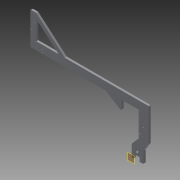
# Autodesk Inventor part: Left Climber Hook_v2
Saved by Autodesk Inventor 2013 (Build 170138000, 138)
## iProperties
Created: 2013-03-16
Part Number: Left Climber Hook_v2
Material: Generic
Document SubType Name: Modeling
Designer: Arpan
Density: 1 g/cm^3
Author: Arpan
Autodesk Inventor part; units mm, degrees
ref_plane "YZ Plane" through (0, 0, 0) normal (1, 0, 0) x (0, 1, 0)
ref_plane "XZ Plane" through (0, 0, 0) normal (0, 1, 0) x (-1, 0, 0)
ref_plane "XY Plane" through (0, 0, 0) normal (0, 0, 1) x (1, 0, 0)
sketch "Sketch1" plane through (0, 0, 0) normal (0, 0, 1) x (1, 0, 0)
  line L0 (0, 0) -> (6.35, 0)
  line L1 (6.35, 0) -> (6.35, 12.7)
  line L2 (6.35, 12.7) -> (25.4, 12.7)
  line L3 (25.4, 12.7) -> (25.4, 0)
  line L4 (25.4, 0) -> (31.75, 0)
  circle A0 centre (15.875, 25.4) radius 4.7815
  line L5 (-323.85, 246.5917) -> (-305.435, 246.5917)
  line L6 (-323.85, 142.875) -> (-83.185, 142.875)
  line L7 (-83.185, 142.875) -> (-37.2427, 114.1611)
  line L8 (-32.385, 142.875) -> (22.225, 142.875)
  line L9 (-32.385, 116.8535) -> (-32.385, 142.875)
  arc A1 (-37.2427, 114.1611) -> (-32.385, 116.8535) centre (-35.56, 116.8535) ccw
  line L10 (-323.85, 168.275) -> (-323.85, 246.5917)
  line L11 (-323.85, 246.5917) -> (-304.8, 246.5917)
  line L12 (-304.8, 229.8394) -> (-304.8, 168.275)
  line L13 (-323.85, 168.275) -> (-323.85, 142.875)
  line L14 (0, 0) -> (0, 38.1)
  line L15 (53.975, -21.4734) -> (53.975, 330.2514) construction
  line L16 (0, 38.1) -> (22.225, 63.5)
  line L17 (22.225, 63.5) -> (22.225, 142.875)
  line L18 (53.975, 63.5) -> (53.975, 168.275)
  line L19 (53.975, 63.5) -> (53.975, 168.275)
  line L20 (22.225, 63.5) -> (22.225, 142.875)
  line L21 (-32.385, 142.875) -> (22.225, 142.875)
  line L22 (-83.185, 142.875) -> (-323.85, 142.875)
  line L23 (31.75, 0) -> (38.1, 0)
  line L24 (38.1, 0) -> (38.1, 38.1)
  line L25 (38.1, 38.1) -> (53.975, 63.5)
  line L26 (38.1, 0) -> (31.75, 0)
  line L27 (-304.8, 246.5917) -> (-213.7569, 168.275)
  line L28 (-233.2314, 168.275) -> (-304.8, 229.8394)
  line L29 (53.975, 168.275) -> (-213.7569, 168.275)
  line L30 (-233.2314, 168.275) -> (-304.8, 168.275)
  line L31 (-304.8, 168.275) -> (-233.2314, 168.275)
  line L32 (-213.7569, 168.275) -> (53.975, 168.275)
  circle A2 centre (-285.75, 149.225) radius 1.5875
  circle A3 centre (-285.75, 161.925) radius 1.5875
  point P0 (-32.385, 111.125)
  point P1 (-359.41, 168.275)
  dimension "d0" = 6.35
  dimension "d1" = 12.7
  dimension "d2" = 19.05
  dimension "d3" = 6.35
  dimension "d4" = 12.7
  dimension "d5" = 9.5631
  dimension "d6" = 12.7
  dimension "d8" = 377.825
  dimension "d17" = 103.7167
  dimension "d19" = 9.525
  dimension "d25" = 31.75
  dimension "d26" = 3.175
  dimension "d27" = 50.8
  dimension "d30" = 19.05
  dimension "d63" = 38.1
  dimension "d68" = 0
  dimension "d69" = 54.61
  dimension "d71" = 22.225
  dimension "d72" = 0
  dimension "d74" = 79.375
  dimension "d75" = 78.3167
  dimension "d76" = 240.665
  dimension "d87" = 6.35
  dimension "d88" = 38.1
  dimension "d89" = 25.4
  dimension "d91" = 25.4
  dimension "d94" = 12.7
  dimension "d95" = 19.05
  dimension "d96" = 25.4
  dimension "d97" = 40.703
  dimension "d98" = 267.7319
  dimension "d109" = 3.175
  dimension "d110" = 3.175
  dimension "d111" = 38.1
  dimension "d112" = 38.1
  dimension "d113" = 6.35
  dimension "d114" = 6.35
  constraints: 66 end point, 10 perpendicular, 9 parallel, 4 centre point, 4 collinear, 4 point on line, 3 horizontal, 2 point on circle, 2 tangent, 2 vertical
  measures "d0" distance of L0.start L0.end
  measures "d1" distance of L0.end L1.end
  measures "d2" distance of L1.end L2.end
  measures "d3" distance of L3.end L4.end
  measures "d4" distance of L2.end L3.end
  measures "d5" diameter of A0
  measures "d6" distance from line of L2 A0.centre
  measures "d8" distance of L29.start L10.start
  measures "d17" distance of L6.start L5.start
  measures "d19" distance from line of L3 A0.centre
  measures "d25" distance of L8.start point (-32.385, 111.125)
  measures "d26" radius of A1
  measures "d27" distance from line of L9 L6.end
  measures "d30" distance of L5.start L11.end
  measures "d63" distance of L0.start L14.end
  measures "d68" distance of L17.end L8.end
  measures "d69" distance of L8.start L8.end
  measures "d71" distance from line of L14 L16.end
  measures "d72" distance of L29.start L18.end
  measures "d74" distance of L16.end L17.end
  measures "d75" distance of L12.end L11.end
  measures "d76" distance of L6.start L6.end
  measures "d87" distance of L4.end L23.end
  measures "d88" distance of L23.end L24.end
  measures "d89" vertical distance of L14.end L16.end
  measures "d91" vertical distance of L18.start L24.end
  measures "d94" distance between parallel lines of L28 L27
  measures "d95" distance between parallel lines of L10 L12
  measures "d96" distance between parallel lines of L6 L30
  measures "d97" angle of L30 L28
  measures "d98" distance of L29.start L27.end
  measures "d109" diameter of A2
  measures "d110" diameter of A3
  measures "d111" distance from line of L13 A3.centre
  measures "d112" distance from line of L13 A2.centre
  measures "d113" distance from line of L6 A2.centre
  measures "d114" distance from line of L30 A3.centre
ref_plane "Work Plane4" through (0, 0, 9.525) normal (0, 0, 1) x (1, 0, 0)
ref_plane "Work Plane3" through (0, 0, 9.525) normal (0, 0, 1) x (1, 0, 0)
extrude "Extrusion9" add sketch "Sketch1" along normal blind 6.35 contours L14 L16 L17 L8 L9 A1 L7 L6 L13 L10 L5 L11 L27 L29 L18 L25 L24 L23 L4 L3 L2 L1 L0 | A2 | A3
sketch "Sketch8" plane through (0, 0, 6.35) normal (0, 0, 1) x (1, 0, 0)
  line L0 (-304.8, 246.5917) -> (-323.85, 246.5917) projected
  line L1 (-323.85, 246.5917) -> (-323.85, 142.875) projected
  circle A0 centre (-309.2958, 218.3215) radius 1.905
  circle A1 centre (-319.405, 195.3091) radius 1.905
  dimension "d101" = 3.81
  dimension "d102" = 3.81
  dimension "d103" = 14.5542
  dimension "d104" = 28.2702
  dimension "d105" = 4.445
  dimension "d106" = 51.2826
  constraints: 2 centre point
  measures "d101" diameter of A0
  measures "d102" diameter of A1
  measures "d103" distance from line of L1 A0.centre
  measures "d104" distance from line of L0 A0.centre
  measures "d105" distance from line of L1 A1.centre
  measures "d106" distance from line of A1.centre L0
extrude "Extrusion10" cut sketch "Sketch8" against normal blind 6.35
sketch "Sketch9" plane through (0, 0, 6.35) normal (0, 0, 1) x (1, 0, 0)
  line L0 (-323.85, 246.5917) -> (-323.85, 142.875) projected
  line L1 (-323.85, 142.875) -> (-83.185, 142.875) projected
  circle A0 centre (-285.75, 155.575) radius 1.5875
  circle A1 centre (-285.75, 147.6375) radius 1.5875
  dimension "d115" = 3.175
  dimension "d116" = 3.175
  dimension "d117" = 38.1
  dimension "d118" = 38.1
  dimension "d119" = 4.7625
  dimension "d124" = 7.9375
  constraints: 2 centre point
  measures "d115" diameter of A0
  measures "d116" diameter of A1
  measures "d117" distance from line of L0 A0.centre
  measures "d118" distance from line of L0 A1.centre
  measures "d119" distance from line of L1 A1.centre
  measures "d124" distance of A1.centre A0.centre
extrude "Extrusion11" cut sketch "Sketch9" against normal blind 6.35
fillet "Fillet8" radius 3.175 14 edges at (-304.8, 246.5917, 3.175) (-323.85, 246.5917, 3.175) (-213.7569, 168.275, 3.175) (53.975, 168.275, 3.175) (53.975, 63.5, 3.175) (38.1, 38.1, 3.175) (0, 0, 3.175) (0, 38.1, 3.175) (22.225, 142.875, 3.175) (22.225, 63.5, 3.175) (-83.185, 142.875, 3.175) (-32.385, 142.875, 3.175) (-323.85, 142.875, 3.175) (-304.8, 229.8394, 3.175)
fillet "Fillet9" radius 3.175 1 edges at (38.1, 0, 3.175)
sketch "Sketch10" plane through (0, 0, 6.35) normal (0, 0, 1) x (1, 0, 0)
  line L0 (-29.21, 142.875) -> (19.05, 142.875) projected
  line L1 (22.225, 139.7) -> (22.225, 64.693) projected
  line L2 (-304.8, 168.275) -> (-304.8, 222.9201) projected
  line L3 (96.2124, 104.775) -> (-86.2445, 104.775) construction
  circle A0 centre (35.5092, 101.6) radius 1.905
  circle A1 centre (25.4, 78.5876) radius 1.905
  point P0 (0, 0)
  dimension "d126" = 38.1
  dimension "d127" = 3.81
  dimension "d128" = 3.81
  dimension "d129" = 10.1092
  dimension "d130" = 23.0124
  dimension "d131" = 3.175
  dimension "d132" = 3.175
  constraints: 2 centre point, 2 end point, 1 perpendicular
  measures "d126" distance between parallel lines of L3 L0
  measures "d127" diameter of A0
  measures "d128" diameter of A1
  measures "d129" horizontal distance of A1.centre A0.centre
  measures "d130" vertical distance of A1.centre A0.centre
  measures "d131" distance from line of L1 A1.centre
  measures "d132" distance from line of L3 A0.centre
extrude "Extrusion12" cut sketch "Sketch10" against normal blind 6.35
body "Solid2"
